Autodesk Fusion 360 part; units mm, degrees
(part 6 of 6)
equation "d5831 = b_Thickness"
equation "d5833 = b_Thickness"
equation "d5835 = b_Thickness"
equation "d5837 = b_Thickness"
equation "d5839 = b_Tool_diameter"
equation "d5840 = b_Tool_diameter"
equation "d5841 = b_Tool_diameter"
equation "d5842 = b_Tool_diameter"
equation "d5843 = b_Tool_diameter"
equation "d5844 = b_Tool_diameter"
equation "d5845 = b_Tool_diameter"
equation "d5846 = b_Tool_diameter"
equation "d5847 = b_Tool_diameter"
equation "d5848 = b_Tool_diameter"
equation "d5850 = b_Thickness"
equation "d5852 = b_Thickness"
equation "d5854 = b_Thickness"
equation "d5856 = b_Thickness"
equation "d5858 = b_Tool_diameter"
equation "d5859 = b_Tool_diameter"
equation "d5860 = b_Tool_diameter"
equation "d5861 = b_Tool_diameter"
equation "d5863 = b_Thickness"
equation "d5865 = b_Thickness"
equation "d5867 = b_Thickness"
equation "d5869 = b_Thickness"
equation "d5871 = b_Thickness"
equation "d5873 = b_Thickness"
equation "d5875 = b_Thickness"
equation "d5877 = b_Thickness"
equation "d5879 = b_Thickness"
equation "d5881 = b_Thickness"
equation "d5883 = b_Tool_diameter"
equation "d5884 = b_Tool_diameter"
equation "d5885 = b_Tool_diameter"
equation "d5886 = b_Tool_diameter"
equation "d5887 = b_Tool_diameter"
equation "d5888 = b_Tool_diameter"
equation "d5889 = b_Tool_diameter"
equation "d5890 = b_Tool_diameter"
equation "d5891 = b_Tool_diameter"
equation "d5892 = b_Tool_diameter"
equation "d5894 = b_Thickness"
equation "d5896 = b_Thickness"
equation "d5898 = b_Thickness"
equation "d5900 = b_Thickness"
equation "d5902 = b_Tool_diameter"
equation "d5903 = b_Tool_diameter"
equation "d5904 = b_Tool_diameter"
equation "d5905 = b_Tool_diameter"
named bodies: "b  stock body", "b top  body", "b top circles cheese body", "b bottom  body", "b bottom circles cheese body", "b front  body", "b front circles cheese body", "b back  body", "b back circles cheese body", "b left  body", "b left circles cheese body", "b right  body", "b right circles cheese body"
